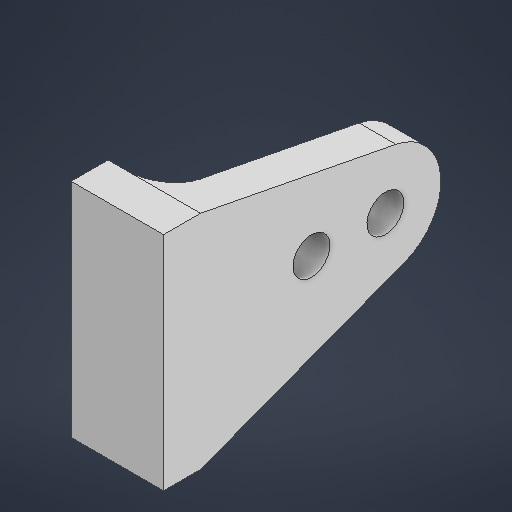
# Autodesk Inventor part: P_Wing_aileron_lever
Saved by Autodesk Inventor 2026 (Build 300175000, 175)
## iProperties
Created: 2025-09-05
Part Number: P_Wing_aileron_lever
Material: Generisch
Document SubType Name: Modeling
Designer: FAL
Density: 1 g/cm^3
Appearance: Vorgabe
Author: FAL
Autodesk Inventor part; units mm, degrees
ref_plane "YZ Plane" through (0, 0, 0) normal (1, 0, 0) x (0, 1, 0)
ref_plane "XZ Plane" through (0, 0, 0) normal (0, 1, 0) x (-1, 0, 0)
ref_plane "XY Plane" through (0, 0, 0) normal (0, 0, 1) x (1, 0, 0)
sketch "Skizze1" plane through (0, 0, 0) normal (1, 0, 0) x (0, 1, 0)
  arc A0 (11.0636, -2.8051) -> (10.5724, 2.9449) centre (10, 0) ccw
  line L0 (11.0636, -2.8051) -> (0, -7)
  line L1 (0, -7) -> (0, 5)
  line L2 (0, 5) -> (10.5724, 2.9449)
  point P0 (0, 0)
  dimension "d0" = 3
  dimension "d1" = 10
  dimension "d2" = 12
  dimension "d3" = 5
  constraints: 6 end point, 2 point on circle, 2 tangent, 1 centre point, 1 horizontal alignment, 1 point on line, 1 vertical
  measures "d0" radius of A0
  measures "d1" distance from line of L1 A0.centre
  measures "d2" distance of L0.end L1.end
  measures "d3" distance of point (0, 0) L1.end
extrude "Extrusion1" add sketch "Skizze1" along normal mid plane 2
sketch "Skizze2" plane through (0, 0, 0) normal (0, 1, 0) x (-1, 0, 0)
  line L0 (-1, 2.9449) -> (-1, 5) projected
  line L1 (-1, 5) -> (4, 5)
  line L2 (4, 5) -> (4, -7)
  line L3 (4, -7) -> (-1, -7)
  line L4 (-1, -7) -> (-1, 5)
  line L5 (1, -7) -> (-1, -7) projected
  point P0 (0, 0)
  point P1 (-1, 2.9449)
  dimension "d6" = 5
  constraints: 8 end point, 2 parallel, 1 collinear, 1 horizontal, 1 perpendicular
  measures "d6" distance between parallel lines of L4 L2
extrude "Extrusion2" add sketch "Skizze2" against normal blind 2
fillet "Rundung1" radius 2 1 edges at (-1, 0, -1)
sketch "Skizze3" plane through (1, 0, 0) normal (1, 0, 0) x (0, 0, -1)
  arc A0 (2.8051, 11.0636) -> (-2.9449, 10.5724) centre (0, 10) ccw projected
  circle A1 centre (0, 10) radius 1
  line L0 (0, 10) -> (0, -2) construction
  line L1 (7, -2) -> (-5, -2) projected
  circle A2 centre (0, 6) radius 1
  point P0 (0, 0)
  dimension "d10" = 2
  dimension "d13" = 4
  constraints: 2 centre point, 2 end point, 2 vertical, 1 coincident, 1 point on line, 2 other
  measures "d10" diameter of A1
  measures "d13" distance of A1.centre A2.centre
extrude "Extrusion3" cut sketch "Skizze3" against normal blind 4.75
